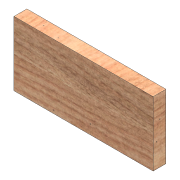
# Autodesk Inventor part: GlassHolder
Saved by Autodesk Inventor 2018 (Build 220112000, 112)
## iProperties
Created: 2020-03-13
Part Number: GlassHolder
Material: Wood (Birch)
Document SubType Name: Modeling
Designer: ottar
Density: 0.55 g/cm^3
Appearance: Birch - Natural Polished
Author: ottar
Autodesk Inventor part; units mm, degrees
ref_plane "YZ Plane" through (0, 0, 0) normal (1, 0, 0) x (0, 1, 0)
ref_plane "XZ Plane" through (0, 0, 0) normal (0, 1, 0) x (-1, 0, 0)
ref_plane "XY Plane" through (0, 0, 0) normal (0, 0, 1) x (1, 0, 0)
sketch "Sketch2" plane through (0, 0, 0) normal (0, 1, 0) x (-1, 0, 0)
  line L0 (0, 0) -> (-215.668, 0)
  line L1 (-215.668, 0) -> (-215.668, -100)
  line L2 (-215.668, -100) -> (0, -100)
  line L3 (0, -100) -> (0, 0)
  dimension "d0" = 215.668
  dimension "d1" = 100
  constraints: 8 end point, 2 parallel, 1 horizontal, 1 perpendicular
  measures "d0" distance of L2.end L1.end
  measures "d1" distance of L1.end L0.end
extrude "Extrusion1" add sketch "Sketch2" along normal blind 20
body "Solid1"
